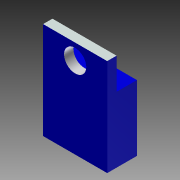
# Autodesk Inventor part: NMOS
Saved by Autodesk Inventor 2012 (Build 160160000, 160)
## iProperties
Created: 2012-04-10
Part Number: NMOS
Material: ABS Plastic
Document SubType Name: Modeling
Designer: admin
Density: 1.06 g/cm^3
Mass: 0.637278 g
Surface Area: 5.43801 cm^2
Volume: 0.601205 cm^3
Author: admin
Autodesk Inventor part; units mm, degrees
ref_plane "YZ Plane" through (0, 0, 0) normal (1, 0, 0) x (0, 1, 0)
ref_plane "XZ Plane" through (0, 0, 0) normal (0, 1, 0) x (-1, 0, 0)
ref_plane "XY Plane" through (0, 0, 0) normal (0, 0, 1) x (1, 0, 0)
sketch "Sketch1" plane through (0, 0, 0) normal (0, 0, 1) x (1, 0, 0)
  line L0 (0, 0) -> (10.414, 0)
  line L1 (10.414, 0) -> (10.414, 10.668)
  line L2 (10.414, 10.668) -> (0, 10.668)
  line L3 (0, 10.668) -> (0, 0)
  dimension "d0" = 10.414
  dimension "d1" = 10.668
  constraints: 8 end point, 2 parallel, 1 horizontal, 1 perpendicular
  measures "d0" distance between parallel lines of L1 L3
  measures "d1" distance between parallel lines of L2 L0
extrude "Extrusion1" add sketch "Sketch1" along normal blind 4.826
sketch "Sketch2" plane through (0, 0, 4.826) normal (0, 0, 1) x (1, 0, 0)
  line L0 (10.414, 10.668) -> (10.414, 0) projected
  line L1 (0, 10.668) -> (10.414, 10.668)
  line L2 (10.414, 10.668) -> (10.414, 15.748)
  line L3 (10.414, 15.748) -> (0, 15.748)
  line L4 (0, 15.748) -> (0, 10.668)
  point P0 (10.414, 5.334)
  dimension "d4" = 5.08
  constraints: 8 end point, 2 parallel, 1 collinear, 1 horizontal, 1 midpoint, 1 perpendicular, 1 point on line
  measures "d4" distance between parallel lines of L1 L3
extrude "Extrusion2" add sketch "Sketch2" against normal blind 1.524
sketch "Sketch3" plane through (0, 0, 3.302) normal (0, 0, -1) x (-1, 0, 0)
  line L0 (0, 0) -> (-10.414, 0) projected
  point P0 (-5.207, 13.208)
  dimension "d7" = 13.208
  measures "d7" distance from line of L0 point (-5.207, 13.208)
hole "Hole1" at (5.207, 13.208, 3.302) direction (0, 0, 1) diameter 3.6068 end through all
body "Solid1"
